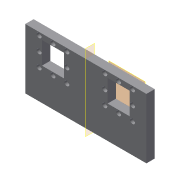
# Autodesk Inventor part: 10_Baseplate_Axiotech_mono
Saved by Autodesk Inventor 2019 (Build 230136000, 136)
## iProperties
Created: 2019-06-11
Part Number: 10_Baseplate_Axiotech_mono
Material: Generic
Document SubType Name: Modeling
Designer: diederichbenedict
Density: 1 g/cm^3
Appearance: Default
Author: diederichbenedict
Autodesk Inventor part; units mm, degrees
ref_plane "YZ Plane" through (0, 0, 0) normal (1, 0, 0) x (0, 1, 0)
ref_plane "XZ Plane" through (0, 0, 0) normal (0, 1, 0) x (-1, 0, 0)
ref_plane "XY Plane" through (0, 0, 0) normal (0, 0, 1) x (1, 0, 0)
ref_plane "Work Plane1" through (0, 0, 0) normal (0, 0, 1) x (1, 0, 0)
ref_plane "Work Plane2" through (0, 0, 0) normal (0, 0, 1) x (1, 0, 0)
sketch "Sketch3" plane through (0, 0, 0) normal (0, 0, 1) x (1, 0, 0)
  circle A0 centre (0, 25) radius 1.95 construction
  circle A1 centre (-25, 0) radius 1.95 construction
  circle A2 centre (-25, -25) radius 1.95 construction
  circle A3 centre (25, 25) radius 1.95 construction
  circle A4 centre (25, -25) radius 1.95 construction
  circle A5 centre (-25, 25) radius 1.95 construction
  circle A6 centre (25, 0) radius 1.95 construction
  circle A7 centre (0, -25) radius 1.95 construction
  line L0 (-28, 30) -> (-30, 28) construction
  line L1 (-30, 28) -> (-30, -28) construction
  line L2 (-30, -28) -> (-28, -30) construction
  line L3 (-28, -30) -> (28, -30) construction
  line L4 (28, -30) -> (30, -28) construction
  line L5 (30, -28) -> (30, 28) construction
  line L6 (30, 28) -> (28, 30) construction
  line L7 (28, 30) -> (-28, 30) construction
  line L8 (30.0525, 30.0525) -> (-59.15, 30.0525)
  line L9 (-59.15, 30.0525) -> (-59.15, -29.9475)
  line L10 (-59.15, -29.9475) -> (30.0525, -29.9475)
  line L11 (30.0525, -29.9475) -> (30.0525, 30.0525)
  line L12 (-59.15, -29.9475) -> (-49.9475, -29.9475)
  line L13 (-49.9475, -29.9475) -> (-49.9475, -69.9475)
  line L14 (-49.9475, -69.9475) -> (-59.15, -69.9475)
  line L15 (-59.15, -69.9475) -> (-59.15, -29.9475)
  circle A8 centre (-59.15, -56.5073) radius 2.9125 construction
  point P0 (0, 0)
  dimension "d6" = 60
  dimension "d8" = 40
  constraints: 16 end point, 4 parallel, 2 horizontal, 2 perpendicular, 1 point on line
  measures "d6" distance of L9.end L8.end
  measures "d8" distance of L12.end L13.end
extrude "Extrusion2" add sketch "Sketch3" along normal blind 12
sketch "Sketch4" plane through (0, 0, 12) normal (0, 0, 1) x (1, 0, 0)
  line L0 (-59.15, 30.0525) -> (-59.15, -69.9475) projected
  line L1 (-59.15, -69.9475) -> (-49.9475, -69.9475) projected
  line L2 (-49.9475, -69.9475) -> (-49.9475, -29.9475) projected
  line L3 (-49.9475, -29.9475) -> (30.0525, -29.9475) projected
  line L4 (30.0525, -29.9475) -> (30.0525, 30.0525) projected
  line L5 (30.0525, 30.0525) -> (-59.15, 30.0525) projected
  line L6 (-49.9475, -69.9475) -> (30.0525, -69.9475)
  line L7 (30.0525, -69.9475) -> (30.0525, -29.9475)
  line L8 (30.0525, -29.9475) -> (-49.9475, -29.9475)
  line L9 (-49.9475, -29.9475) -> (-49.9475, -69.9475)
  point P0 (0, 0)
  constraints: 8 end point, 2 parallel, 1 horizontal, 1 perpendicular
extrude "Extrusion3" add sketch "Sketch4" along normal blind 3
sketch "Sketch5" plane through (0, 0, 15) normal (0, 0, 1) x (1, 0, 0)
  line L0 (-59.15, -69.9475) -> (30.0525, -69.9475) projected
  line L1 (30.0525, -69.9475) -> (30.0525, 30.0525) projected
  line L2 (30.0525, 30.0525) -> (-59.15, 30.0525) projected
  line L3 (-59.15, 30.0525) -> (-59.15, -69.9475) projected
  line L4 (-59.15, -69.9475) -> (-49.9475, -69.9475) projected
  line L5 (-59.15, -69.9475) -> (50.85, -69.9475)
  line L6 (50.85, -69.9475) -> (50.85, -78.3535)
  line L7 (50.85, -78.3535) -> (-59.15, -78.3535)
  line L8 (-59.15, -78.3535) -> (-59.15, -69.9475)
  line L9 (50.85, -78.3535) -> (54.85, -78.3535)
  line L10 (54.85, -78.3535) -> (54.85, -24.0007)
  line L11 (54.85, -24.0007) -> (50.85, -24.0007)
  line L12 (50.85, -24.0007) -> (50.85, -78.3535)
  point P0 (0, 0)
  dimension "d13" = 110
  dimension "d14" = 8.406
  dimension "d15" = 4
  dimension "d16" = 54.353
  constraints: 16 end point, 4 parallel, 2 horizontal, 2 perpendicular
  measures "d13" distance of L6.end L7.end
  measures "d15" distance of L11.end L10.end
extrude "Extrusion4" add sketch "Sketch5" against normal up to surface (15 mm away) contours L0 L5 L6 L7 L8
sketch "Sketch6" plane through (0, 0, 15) normal (0, 0, 1) x (1, 0, 0)
  line L0 (30.0525, -69.9475) -> (30.0525, 30.0525) projected
  line L1 (30.0525, 30.0525) -> (-59.15, 30.0525) projected
  line L2 (-59.15, 30.0525) -> (-59.15, -78.3535) projected
  line L3 (-59.15, -78.3535) -> (50.85, -78.3535) projected
  circle A0 centre (0, 25) radius 1.95 projected
  circle A1 centre (-25, 0) radius 1.95 projected
  circle A2 centre (-25, -25) radius 1.95 projected
  circle A3 centre (25, 25) radius 1.95 projected
  circle A4 centre (25, -25) radius 1.95 projected
  circle A5 centre (-25, 25) radius 1.95 projected
  circle A6 centre (25, 0) radius 1.95 projected
  circle A7 centre (0, -25) radius 1.95 projected
  line L4 (-28, 30) -> (-30, 28) projected
  line L5 (-30, 28) -> (-30, -28) projected
  line L6 (-30, -28) -> (-28, -30) projected
  line L7 (-28, -30) -> (28, -30) projected
  line L8 (28, -30) -> (30, -28) projected
  line L9 (30, -28) -> (30, 28) projected
  line L10 (30, 28) -> (28, 30) projected
  line L11 (28, 30) -> (-28, 30) projected
  line L12 (50.85, -78.3535) -> (50.85, -69.9475) projected
  line L13 (50.85, -69.9475) -> (30.0525, -69.9475) projected
  point P0 (0, 0)
  constraints: 1 coincident
hole "Hole1" at (25, 25, 15) at (0, 25, 15) at (-25, 25, 15) at (-25, 0, 15) at (-25, -25, 15) at (0, -25, 15) at (25, -25, 15) at (25, 0, 15) direction (0, 0, -1) diameter 4.2 end through all counterbore diameter 9 counterbore depth 5
sketch "Sketch7" plane through (30.0525, -29.9475, 0) normal (1, 0, 0) x (0, 0, -1)
  line L0 (-10, 34.4475) -> (-10, 25.4475) projected
  line L1 (0, 0) -> (0, 60) projected
  line L2 (0, 60) -> (-15, 60) projected
  line L3 (-15, -40) -> (-15, 60) projected
  line L4 (-12, -40) -> (-12, 0) projected
  line L5 (0, 0) -> (-12, 0) projected
  line L6 (-12, -40) -> (-15, -40) projected
  point P0 (0, 29.9475)
extrude "Extrusion5" add sketch "Sketch7" along normal blind 10
sketch "Sketch8" plane through (40.0525, -29.9475, 0) normal (1, 0, 0) x (0, 0, -1)
  line L0 (0, 0) -> (0, 60) projected
  line L1 (0, 60) -> (-15, 60) projected
  line L2 (-15, 60) -> (-15, -40) projected
  line L3 (-12, -40) -> (-12, 0) projected
  line L4 (-12, 0) -> (0, 0) projected
  line L5 (0, 0) -> (-12, 0)
  line L6 (-12, 0) -> (-12, -40)
  line L7 (-12, -40) -> (0, -40)
  line L8 (0, -40) -> (0, 0)
  line L9 (-12, -40) -> (-15, -40) projected
  point P0 (0, 29.9475)
  constraints: 8 end point, 2 parallel, 1 horizontal, 1 perpendicular
extrude "Extrusion6" add sketch "Sketch8" along normal blind 10
sketch "Sketch10" plane through (0, 0, 0) normal (0, 0, -1) x (-1, 0, 0)
  line L0 (49.9475, -29.9475) -> (-40.0525, -29.9475) construction
  line L1 (49.9475, -69.9475) -> (49.9475, -29.9475) construction
  line L2 (49.9475, -69.9475) -> (-40.0525, -69.9475) construction
  line L3 (-40.0525, -69.9475) -> (-40.0525, -29.9475) construction
  circle A0 centre (-25, -25) radius 2.1 construction
  circle A1 centre (25, -25) radius 2.1 construction
  circle A2 centre (25, 25) radius 2.1 construction
  circle A3 centre (-25, 25) radius 2.1 construction
  circle A4 centre (0, 25) radius 2.1 construction
  circle A5 centre (25, 0) radius 2.1 construction
  circle A6 centre (0, -25) radius 2.1 construction
  circle A7 centre (-25, 0) radius 2.1 construction
  line L4 (-50.0525, 30.0525) -> (59.15, 30.0525) construction
  line L5 (-50.0525, -69.9475) -> (-50.0525, 30.0525) construction
  line L6 (-50.85, -78.3535) -> (59.15, -78.3535) construction
  line L7 (59.15, 30.0525) -> (59.15, -78.3535) construction
  line L8 (39, -67) -> (34, -67) construction
  line L9 (34, -71) -> (34, -67) construction
  line L10 (34, -71) -> (39, -71) construction
  line L11 (39, -67) -> (39, -71) construction
  line L12 (28.1949, -69.9475) -> (49.9475, -69.9475)
  line L13 (49.9475, -69.9475) -> (49.9475, -73.7985)
  line L14 (49.9475, -73.7985) -> (28.1949, -73.7985)
  line L15 (28.1949, -73.7985) -> (28.1949, -69.9475)
  line L16 (-50.0525, -69.9475) -> (-50.85, -69.9475) projected
  line L17 (-50.85, -69.9475) -> (-50.85, -78.3535) projected
  point P0 (0, 0)
  constraints: 8 end point, 2 parallel, 1 horizontal, 1 perpendicular, 1 point on line
extrude "Extrusion8" cut sketch "Sketch10" against normal up to surface (12 mm away)
sketch "Sketch15" plane through (0, 0, 0) normal (0, 0, -1) x (-1, 0, 0)
  circle A0 centre (0, 0) radius 7.5 projected
  line L0 (20, -20) -> (-20, -20)
  line L1 (-20, -20) -> (-20, 20)
  line L2 (-20, 20) -> (20, 20)
  line L3 (20, 20) -> (20, -20)
  line L4 (20, -20) -> (-20, 20) construction
  line L5 (-20, -20) -> (20, 20) construction
  point P0 (0, 0)
  dimension "d52" = 40
  dimension "d53" = 40
  constraints: 12 end point, 2 midpoint, 2 parallel, 1 horizontal, 1 perpendicular
  measures "d52" distance of L1.end L2.end
  measures "d53" distance of L0.end L1.end
extrude "Extrusion10" cut sketch "Sketch15" against normal through all contours A0 | L0 L1 L2 L3
mirror "Mirror2" about plane through (-59.15, -29.9475, 0) normal (-1, 0, 0) of "Extrusion2", "Extrusion3", "Extrusion4", "Hole1", "Extrusion5", "Extrusion6", "Extrusion8", "Extrusion10"
sketch "Sketch20" plane through (0, 0, 0) normal (0, 0, -1) x (-1, 0, 0)
  circle A0 centre (59.15, -56.5073) radius 2.9125 projected
  line L0 (14, -48.5) -> (-39, -48.5)
  line L1 (14, -53.5) -> (-39, -53.5)
  line L2 (-21.1695, -50.8251) -> (110.767, -50.8251)
  line L3 (52.1305, -46.7848) -> (66.1268, -46.7848)
  line L4 (66.1268, -46.7848) -> (59.1286, -58.9059)
  line L5 (59.1286, -58.9059) -> (52.1305, -46.7848)
  point P0 (0, 0)
  point P1 (59.1286, -50.8251)
  dimension "d75" = 180
  constraints: 12 end point, 3 horizontal, 1 point on line, 11 other
  measures "d75" angle of L3 L0
hole "Hole6" at (-52.1305, -46.7848, 0) at (-66.1268, -46.7848, 0) at (-59.1286, -58.9059, 0) direction (0, 0, 1) diameter 2.8 end through all
body "Solid2"
